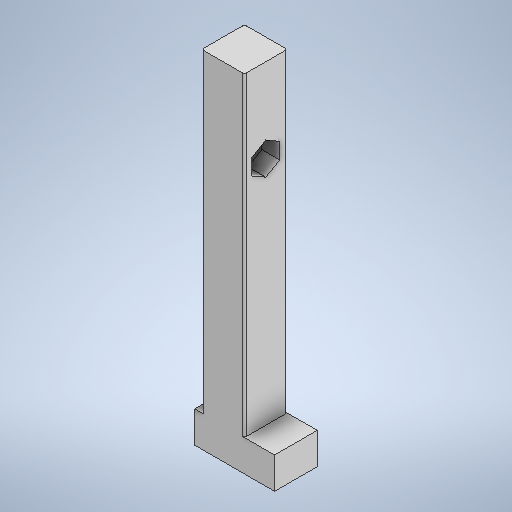
# Autodesk Inventor part: shaft4V1
Saved by Autodesk Inventor 2025.2 (Build 292293000, 293)
## iProperties
Created: 2025-04-02
Part Number: shaft4V1
Material: Generic
Document SubType Name: Modeling
Designer: patrickandersen
Density: 1 g/cm^3
Appearance: Default
Author: patrickandersen
Autodesk Inventor part; units mm, degrees
ref_plane "YZ Plane" through (0, 0, 0) normal (1, 0, 0) x (0, 1, 0)
ref_plane "XZ Plane" through (0, 0, 0) normal (0, 1, 0) x (-1, 0, 0)
ref_plane "XY Plane" through (0, 0, 0) normal (0, 0, 1) x (1, 0, 0)
sketch "Sketch1" plane through (0, 0, 0) normal (0, 1, 0) x (-1, 0, 0)
  line L0 (5.4777, 10.4253) -> (-14.8723, 10.4253)
  line L1 (-14.8723, 10.4253) -> (-14.8723, -9.9247)
  line L2 (-14.8723, -9.9247) -> (5.4777, -9.9247)
  line L3 (5.4777, -9.9247) -> (5.4777, 10.4253)
  point P0 (0, 0)
  dimension "d0" = 20.35
  dimension "d1" = 20.35
  constraints: 8 end point, 2 parallel, 1 horizontal, 1 perpendicular
  measures "d0" distance of L2.end L0.start
  measures "d1" distance of L0.start L0.end
extrude "Extrusion1" add sketch "Sketch1" along normal blind 150
fillet "Fillet1" radius 1 4 edges at (14.8723, 75, 10.4253) (14.8723, 75, -9.9247) (-5.4777, 75, 10.4253) (-5.4777, 75, -9.9247)
sketch "Sketch2" plane through (14.8723, 0, 9.4253) normal (1, 0, 0) x (0, 0, -1)
  line L0 (9.175, 102.3501) -> (2.55, 106.1751)
  line L1 (2.55, 106.1751) -> (2.55, 113.8249)
  line L2 (2.55, 113.8249) -> (9.175, 117.6499)
  line L3 (9.175, 117.6499) -> (15.8, 113.8249)
  line L4 (15.8, 113.8249) -> (15.8, 106.1751)
  line L5 (15.8, 106.1751) -> (9.175, 102.3501)
  line L6 (18.35, 150) -> (18.35, 0) projected
  line L7 (0, 150) -> (18.35, 150) projected
  line L8 (0, 0) -> (0, 150) projected
  line L9 (0, 0) -> (18.35, 0) projected
  line L10 (-1, 150) -> (-1, 0) projected
  point P0 (9.4253, 0)
  point P1 (9.175, 110)
  dimension "d5" = 13.25
  dimension "d6" = 0
  dimension "d37" = 110
  dimension "d39" = 40
  dimension "d40" = 10.175
  constraints: 12 end point, 13 other
  measures "d5" distance between parallel lines of L3 L0
  measures "d6" angle of L6 L4
  measures "d37" distance from line of L9 point (9.175, 110)
  measures "d39" distance from line of L7 point (9.175, 110)
  measures "d40" distance from line of L10 point (9.175, 110)
extrude "Extrusion2" cut sketch "Sketch2" against normal blind 8.5 contours L0 L1 L2 L3 L4 L5
sketch "Sketch3" plane through (-5.4777, 0, -8.9247) normal (-1, 0, 0) x (0, 0, 1)
  circle A0 centre (9.175, 110) radius 9.25
  line L0 (0, 150) -> (18.35, 150) projected
  line L1 (19.35, 0) -> (19.35, 150) projected
  line L2 (0, 0) -> (18.35, 0) projected
  point P0 (8.9247, 0)
  dimension "d12" = 18.5
  dimension "d13" = 10.175
  dimension "d38" = 110
  constraints: 1 centre point
  measures "d12" diameter of A0
  measures "d13" distance from line of L1 A0.centre
  measures "d38" distance from line of L2 A0.centre
hole "Hole1" at (-5.4777, 110, 0.2503) direction (1, 0, 0) diameter 8.5 depth 40 counterbore diameter 18.5 counterbore depth 6
sketch "Sketch4" plane through (0, 0, 0) normal (0, -1, 0) x (1, 0, 0)
  line L0 (29.2223, -9.9247) -> (-8.8277, -9.9247)
  line L1 (-8.8277, -9.9247) -> (-8.8277, 10.4253)
  line L2 (-8.8277, 10.4253) -> (29.2223, 10.4253)
  line L3 (29.2223, 10.4253) -> (29.2223, -9.9247)
  line L4 (13.8723, -9.9247) -> (-4.4777, -9.9247) projected
  line L5 (14.8723, 9.4253) -> (14.8723, -8.9247) projected
  line L6 (-5.4777, -8.9247) -> (-5.4777, 9.4253) projected
  point P0 (0, 0)
  dimension "d22" = 20.35
  dimension "d23" = 0
  dimension "d25" = 3.35
  dimension "d36" = 14.35
  constraints: 8 end point, 2 parallel, 1 horizontal, 1 perpendicular
  measures "d22" distance of L0.end L1.end
  measures "d23" distance between parallel lines of L4 L0
  measures "d25" distance between parallel lines of L6 L1
  measures "d36" distance between parallel lines of L5 L3
extrude "Extrusion3" add sketch "Sketch4" along normal blind 15
body "Solid1"
